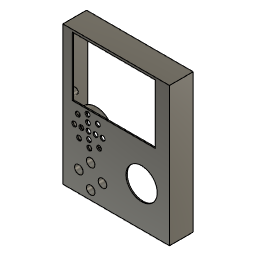
front2 (Autodesk Fusion 360 design; units mm, degrees)
Autodesk Fusion 360 part; units mm, degrees
sketch "Sketch1" plane through (0, 0, 0) normal (0, 1, 0) x (1, 0, 0)
  line L0 (-88, -115.2) -> (-2, -115.2)
  line L1 (-2, -115.2) -> (-2, -65.2)
  line L2 (-2, -65.2) -> (-88, -65.2)
  line L3 (-88, -65.2) -> (-88, -115.2)
  line L4 (-12, -115.2) -> (-82, -115.2)
  line L5 (-82, -115.2) -> (-82, -65.2)
  line L6 (-82, -65.2) -> (-12, -65.2)
  line L7 (-12, -65.2) -> (-12, -115.2)
  circle A0 centre (-85, -112.2) radius 1.5
  circle A1 centre (-85, -68.2) radius 1.5
  circle A2 centre (-8.8, -112.2) radius 1.5
  circle A3 centre (-8.8, -68.2) radius 1.5
  line L8 (-72, -33) -> (-61, -33)
  line L9 (-61, -33) -> (-61, -22)
  line L10 (-61, -22) -> (-72, -22)
  line L11 (-72, -22) -> (-72, -33)
  line L12 (-62, -23) -> (-51, -23)
  line L13 (-51, -23) -> (-51, -12)
  line L14 (-51, -12) -> (-62, -12)
  line L15 (-62, -12) -> (-62, -23)
  line L16 (-61, -13) -> (-72, -13)
  line L17 (-72, -13) -> (-72, -2)
  line L18 (-72, -2) -> (-61, -2)
  line L19 (-61, -2) -> (-61, -13)
  line L20 (-71, -23) -> (-82, -23)
  line L21 (-82, -23) -> (-82, -12)
  line L22 (-82, -12) -> (-71, -12)
  line L23 (-71, -12) -> (-71, -23)
  line L24 (-61, -22) -> (-52, -22)
  line L25 (-52, -22) -> (-52, -13)
  line L26 (-52, -13) -> (-61, -13)
  line L27 (-61, -13) -> (-61, -22)
  line L28 (-71, -23) -> (-62, -23)
  line L29 (-62, -23) -> (-62, -32)
  line L30 (-62, -32) -> (-71, -32)
  line L31 (-71, -32) -> (-71, -23)
  line L32 (-72, -22) -> (-81, -22)
  line L33 (-81, -22) -> (-81, -13)
  line L34 (-81, -13) -> (-72, -13)
  line L35 (-72, -13) -> (-72, -22)
  line L36 (-71, -12) -> (-62, -12)
  line L37 (-62, -12) -> (-62, -3)
  line L38 (-62, -3) -> (-71, -3)
  line L39 (-71, -3) -> (-71, -12)
  circle A4 centre (-66.5, -7.5) radius 3.6
  circle A5 centre (-76.5, -17.5) radius 3.6
  circle A6 centre (-56.5, -17.5) radius 3.6
  circle A7 centre (-66.5, -27.5) radius 3.6
  circle A8 centre (-73.5, -10.5) radius 1.5
  circle A9 centre (-59.5, -24.5) radius 1.5
  circle A10 centre (-59.5, -24.5) radius 2.5
  circle A11 centre (-73.5, -10.5) radius 2.5
  line L40 (-73.5048, -8) -> (-72, -8)
  line L41 (-72, -8) -> (-72, -8.5)
  line L42 (-72, -8.5) -> (-73.5048, -8.5)
  line L43 (-73.5048, -8.5) -> (-73.5048, -8)
  line L44 (-76, -10.5053) -> (-75.5, -10.5053)
  line L45 (-75.5, -10.5053) -> (-75.5, -12)
  line L46 (-75.5, -12) -> (-76, -12)
  line L47 (-76, -12) -> (-76, -10.5053)
  line L48 (-57, -24.4959) -> (-57.5, -24.4959)
  line L49 (-57.5, -24.4959) -> (-57.5, -23)
  line L50 (-57.5, -23) -> (-57, -23)
  line L51 (-57, -23) -> (-57, -24.4959)
  line L52 (-59.4955, -27) -> (-61, -27)
  line L53 (-61, -27) -> (-61, -26.5)
  line L54 (-61, -26.5) -> (-59.4955, -26.5)
  line L55 (-59.4955, -26.5) -> (-59.4955, -27)
  circle A12 centre (-23.5, -33.6) radius 13.2
  circle A13 centre (-68.4, -49.6) radius 14.1
  circle A14 centre (-68.4, -49.6) radius 14.6
  circle A15 centre (-68.4, -49.6) radius 2
  circle A16 centre (-69.1779, -61.5748) radius 2
  circle A17 centre (-68.8197, -55.5853) radius 2
  circle A18 centre (-60.4826, -58.6175) radius 2
  circle A19 centre (-56.4253, -50.3779) radius 2
  circle A20 centre (-59.3825, -41.6826) radius 2
  circle A21 centre (-67.6221, -37.6252) radius 2
  circle A22 centre (-76.3174, -40.5825) radius 2
  circle A23 centre (-80.3748, -48.8221) radius 2
  circle A24 centre (-77.4175, -57.5174) radius 2
  circle A25 centre (-62.4147, -50.0197) radius 2
  circle A26 centre (-67.9803, -43.6147) radius 2
  circle A27 centre (-74.3853, -49.1803) radius 2
  circle A28 centre (-51.3037, -49.9525) radius 2.5
  circle A29 centre (-51.3037, -49.9525) radius 1.5
  circle A30 centre (-85.5, -49.572) radius 2.5
  circle A31 centre (-85.5, -49.572) radius 1.5
  line L56 (-85.6266, -52.0687) -> (-83, -52.0687)
  line L57 (-83, -52.0687) -> (-83, -49.5761)
  line L58 (-83, -49.5761) -> (-85.6266, -49.5761)
  line L59 (-85.6266, -49.5761) -> (-85.6266, -52.0687)
  line L60 (-82.7898, -52.0687) -> (-83, -52.0687)
  line L61 (-83, -52.0687) -> (-83, -49.5761)
  line L62 (-83, -49.5761) -> (-82.7898, -49.5761)
  line L63 (-82.7898, -49.5761) -> (-82.7898, -52.0687)
  line L64 (-85.3581, -47.076) -> (-82.7898, -47.076)
  line L65 (-82.7898, -47.076) -> (-82.7898, -49.5761)
  line L66 (-82.7898, -49.5761) -> (-85.3581, -49.5761)
  line L67 (-85.3581, -49.5761) -> (-85.3581, -47.076)
  line L68 (-51.4135, -52.4501) -> (-53.8031, -52.4501)
  line L69 (-53.8031, -52.4501) -> (-53.8031, -49.901)
  line L70 (-53.8031, -49.901) -> (-51.4135, -49.901)
  line L71 (-51.4135, -49.901) -> (-51.4135, -52.4501)
  line L72 (-53.8031, -49.901) -> (-51.1807, -49.901)
  line L73 (-51.1807, -49.901) -> (-51.1807, -47.4555)
  line L74 (-51.1807, -47.4555) -> (-53.8031, -47.4555)
  line L75 (-53.8031, -47.4555) -> (-53.8031, -49.901)
  line L76 (-53.9584, -47.4555) -> (-53.8031, -47.4555)
  line L77 (-53.8031, -47.4555) -> (-53.8031, -49.901)
  line L78 (-53.8031, -49.901) -> (-53.9584, -49.901)
  line L79 (-53.9584, -49.901) -> (-53.9584, -47.4555)
  line L80 (-54.0809, -52.4501) -> (-53.8031, -52.4501)
  line L81 (-53.8031, -52.4501) -> (-53.8031, -49.901)
  line L82 (-53.8031, -49.901) -> (-54.0809, -49.901)
  line L83 (-54.0809, -49.901) -> (-54.0809, -52.4501)
  line L84 (-90, -117.2) -> (0, -117.2)
  line L85 (0, -117.2) -> (0, 0)
  line L86 (0, 0) -> (-90, 0)
  line L87 (-90, 0) -> (-90, -117.2)
  line L88 (-89, -116.2) -> (-1, -116.2)
  line L89 (-1, -116.2) -> (-1, -1)
  line L90 (-1, -1) -> (-89, -1)
  line L91 (-89, -1) -> (-89, -116.2)
  circle A32 centre (-85, -112.2) radius 2.5
  circle A33 centre (-85, -68.2) radius 2.5
  circle A34 centre (-8.8, -68.2) radius 2.5
  circle A35 centre (-8.8, -112.2) radius 2.5
  dimension "d1" = 86
  dimension "d2" = 50
  dimension "d3" = 70
  dimension "d4" = 50
  dimension "d5" = 10
  dimension "d6" = 3
  dimension "d7" = 3
  dimension "d8" = 3
  dimension "d9" = 3
  dimension "d10" = 3
  dimension "d11" = 3
  dimension "d12" = 3
  dimension "d13" = 3
  dimension "d14" = 6.8
  dimension "d15" = 3
  dimension "d16" = 6.8
  dimension "d17" = 3
  dimension "d18" = 11
  dimension "d19" = 11
  dimension "d20" = 11
  dimension "d21" = 11
  dimension "d22" = 11
  dimension "d23" = 11
  dimension "d24" = 11
  dimension "d25" = 11
  dimension "d26" = 1
  dimension "d27" = 1
  dimension "d28" = 1
  dimension "d29" = 1
  dimension "d30" = 1
  dimension "d31" = 1
  dimension "d32" = 9
  dimension "d33" = 9
  dimension "d34" = 9
  dimension "d35" = 9
  dimension "d36" = 9
  dimension "d37" = 9
  dimension "d38" = 9
  dimension "d39" = 9
  dimension "d40" = 7.2
  dimension "d41" = 7.2
  dimension "d42" = 7.2
  dimension "d43" = 7.2
  dimension "d44" = 4.5
  dimension "d45" = 4.5
  dimension "d46" = 4.5
  dimension "d47" = 4.5
  dimension "d48" = 4.5
  dimension "d49" = 4.5
  dimension "d50" = 4.5
  dimension "d51" = 4.5
  dimension "d52" = 3
  dimension "d53" = 3
  dimension "d54" = 1.5
  dimension "d55" = 1.5
  dimension "d56" = 1.5
  dimension "d57" = 1.5
  dimension "d58" = 5
  dimension "d59" = 5
  dimension "d60" = 26.4
  dimension "d61" = 28.2
  dimension "d62" = 29.2
  dimension "d63" = 4
  dimension "d64" = 4
  dimension "d65" = 12
  dimension "d66" = 4
  dimension "d67" = 6
  dimension "d69" = 360
  dimension "d71" = 360
  dimension "d72" = 5
  dimension "d73" = 3
  dimension "d74" = 5
  dimension "d75" = 3
  dimension "d76" = 17.1
  dimension "d77" = 17.0964
  dimension "d78" = 15.6
  dimension "d79" = 2.5
  dimension "d80" = 16.6
  dimension "d81" = 7.4
  dimension "d83" = 27.5
  dimension "d85" = 31.6
  dimension "d86" = 2
  dimension "d87" = 2
  dimension "d88" = 2
  dimension "d89" = 2
  dimension "d90" = 1
  dimension "d91" = 1
  dimension "d92" = 1
  dimension "d93" = 1
  dimension "d98" = 5
  dimension "d99" = 5
  dimension "d100" = 5
  dimension "d101" = 5
  constraint horizontal L0
  constraint vertical L1
  constraint horizontal L2
  constraint vertical L3
  constraint horizontal L4
  constraint vertical L5
  constraint horizontal L6
  constraint vertical L7
  constraint coincident L0 L4.start
  constraint horizontal L8
  constraint vertical L9
  constraint horizontal L10
  constraint vertical L11
  constraint horizontal L12
  constraint vertical L13
  constraint horizontal L14
  constraint vertical L15
  constraint horizontal L16
  constraint vertical L17
  constraint horizontal L18
  constraint vertical L19
  constraint horizontal L20
  constraint vertical L21
  constraint horizontal L22
  constraint vertical L23
  constraint horizontal L24
  constraint vertical L25
  constraint horizontal L26
  constraint vertical L27
  constraint horizontal L28
  constraint vertical L29
  constraint horizontal L30
  constraint vertical L31
  constraint horizontal L32
  constraint vertical L33
  constraint horizontal L34
  constraint vertical L35
  constraint horizontal L36
  constraint vertical L37
  constraint horizontal L38
  constraint vertical L39
  constraint concentric A9 A10
  constraint concentric A8 A11
  constraint horizontal L40
  constraint vertical L41
  constraint horizontal L42
  constraint vertical L43
  constraint coincident A11 L41.end
  constraint coincident L17 L41.end
  constraint coincident A11 L40.start
  constraint horizontal L44
  constraint vertical L45
  constraint horizontal L46
  constraint vertical L47
  constraint coincident A11 L45.end
  constraint coincident L22 L45.end
  constraint coincident A11 L44.start
  constraint horizontal L48
  constraint vertical L49
  constraint horizontal L50
  constraint vertical L51
  constraint coincident L12 L49.end
  constraint coincident A10 L49.end
  constraint coincident A10 L48.start
  constraint horizontal L52
  constraint vertical L53
  constraint horizontal L54
  constraint vertical L55
  constraint coincident A10 L53.end
  constraint coincident L9 L53.end
  constraint coincident A10 L52.start
  constraint concentric A13 A14
  constraint concentric A13 A15
  constraint concentric A28 A29
  constraint tangent A14 A28
  constraint concentric A30 A31
  constraint tangent A14 A30
  constraint horizontal L56
  constraint vertical L57
  constraint horizontal L58
  constraint vertical L59
  constraint coincident A30 L57.end
  constraint coincident A14 L57.end
  constraint coincident A30 L56.start
  constraint horizontal L60
  constraint vertical L61
  constraint horizontal L62
  constraint vertical L63
  constraint coincident A14 L60.start
  constraint horizontal L64
  constraint vertical L65
  constraint horizontal L66
  constraint vertical L67
  constraint coincident A30 L64.start
  constraint horizontal L68
  constraint vertical L69
  constraint horizontal L70
  constraint vertical L71
  constraint coincident A28 L69.end
  constraint coincident A14 L69.end
  constraint coincident A28 L68.start
  constraint horizontal L72
  constraint vertical L73
  constraint horizontal L74
  constraint vertical L75
  constraint coincident A28 L73.end
  constraint horizontal L76
  constraint vertical L77
  constraint horizontal L78
  constraint vertical L79
  constraint coincident A14 L76.start
  constraint horizontal L80
  constraint vertical L81
  constraint horizontal L82
  constraint vertical L83
  constraint coincident A14 L80.start
  constraint coincident L68.end L80
  constraint coincident L74.end L76
  constraint coincident L56.end L60
  constraint horizontal L84
  constraint vertical L85
  constraint horizontal L86
  constraint vertical L87
  constraint horizontal L88
  constraint vertical L89
  constraint horizontal L90
  constraint vertical L91
  constraint concentric A0 A32
  constraint concentric A1 A33
  constraint concentric A3 A34
  constraint concentric A2 A35
  constraint coincident L85.end L86.start
  measures "d1" distance of L0.start L0.end
  measures "d2" distance of L0.start L2.end
  measures "d3" distance of L4.start L4.end
  measures "d4" distance of L4.start L6.end
  measures "d5" distance of L1 L7
  measures "d6" diameter of A0
  measures "d7" diameter of A1
  measures "d8" diameter of A2
  measures "d9" diameter of A3
  measures "d10" distance of L3 A1.centre
  measures "d11" distance of L2 A1.centre
  measures "d12" distance of L3 A0.centre
  measures "d13" distance of L0 A0.centre
  measures "d14" distance of L1 A2.centre
  measures "d15" distance of L0 A2.centre
  measures "d16" distance of L1 A3.centre
  measures "d17" distance of L2 A3.centre
  measures "d18" distance of L8.start L8.end
  measures "d19" distance of L8.start L10.end
  measures "d20" distance of L12.start L12.end
  measures "d21" distance of L12.start L14.end
  measures "d22" distance of L16.start L16.end
  measures "d23" distance of L16.start L18.end
  measures "d24" distance of L20.start L20.end
  measures "d25" distance of L20.start L22.end
  measures "d26" distance of L16 L22
  measures "d27" distance of L17 L23
  measures "d28" distance of L15 L19
  measures "d29" distance of L14 L16
  measures "d30" distance of L10 L12
  measures "d31" distance of L9 L15
  measures "d32" distance of L9.end L24.end
  measures "d33" distance of L9.end L16.start
  measures "d34" distance of L20.start L12.start
  measures "d35" distance of L20.start L30.end
  measures "d36" distance of L10.end L32.end
  measures "d37" distance of L10.end L16.end
  measures "d38" distance of L22.end L14.end
  measures "d39" distance of L22.end L38.end
  measures "d40" diameter of A4
  measures "d41" diameter of A5
  measures "d42" diameter of A6
  measures "d43" diameter of A7
  measures "d44" distance of L39 A4.centre
  measures "d45" distance of L38 A4.centre
  measures "d46" distance of L26 A6.centre
  measures "d47" distance of L25 A6.centre
  measures "d48" distance of L34 A5.centre
  measures "d49" distance of L35 A5.centre
  measures "d50" distance of L29 A7.centre
  measures "d51" distance of L28 A7.centre
  measures "d52" diameter of A8
  measures "d53" diameter of A9
  measures "d54" distance of L22 A8.centre
  measures "d55" distance of L17 A8.centre
  measures "d56" distance of L12 A9.centre
  measures "d57" distance of L9 A9.centre
  measures "d58" diameter of A10
  measures "d59" diameter of A11
  measures "d60" diameter of A12
  measures "d61" diameter of A13
  measures "d62" diameter of A14
  measures "d63" diameter of A15
  measures "d64" diameter of A16
  measures "d65" distance of A13.centre A16.centre
  measures "d66" diameter of A17
  measures "d67" distance of A13.centre A17.centre
  measures "d72" diameter of A28
  measures "d73" diameter of A29
  measures "d74" diameter of A30
  measures "d75" diameter of A31
  measures "d76" horizontal distance of A13.centre A30.centre
  measures "d77" horizontal distance of A13.centre A28.centre
  measures "d78" distance of L2 A13.centre
  measures "d79" distance of L3 A30.centre
  measures "d80" distance of L8 A13.centre
  measures "d81" distance of L9 A13.centre
  measures "d83" distance of L13 A12.centre
  measures "d85" distance of L2 A12.centre
  measures "d86" distance of L18 L86
  measures "d87" distance of L3 L87
  measures "d88" distance of L4 L84
  measures "d89" distance of L1 L85
  measures "d90" distance of L85 L89
  measures "d91" distance of L84 L88
  measures "d92" distance of L87 L91
  measures "d93" distance of L86 L90
  measures "d98" diameter of A32
  measures "d99" diameter of A33
  measures "d100" diameter of A34
  measures "d101" diameter of A35
extrude "Extrude1" add sketch "Sketch1" against normal blind 1 contours L0 L2 L3 L5 | L0 L1 L2 L7 | A0 | A1 | A2 | A3 | L8 L9 L11 L20 L29 L30 L31 A10 L53 | L17 A11 L40 L41 | L9 A10 L52 L53 | L11 L20 L21 L22 L32 L33 L34 A11 L46 | L10 L11 L20 L23 | L10 L16 L23 L35 | L32 L33 L34 L35 | L10 L15 L23 L28 | L28 L29 L30 L31 | L9 L12 A10 | A10 L54 L55 | L9 L12 A9 A10 L48 L49 L54 L55 | L10 L15 L16 L23 | L16 L17 L22 L23 A11 | L17 L34 A11 | L9 L10 L12 L15 A10 | L12 L29 A10 | L9 L12 A9 | A9 | L10 L15 L16 L27 | L15 L16 L23 L36 | L17 L22 A11 | L17 L22 A11 | L9 L12 A10 | L22 A11 L46 L47 | L9 L12 A10 | A10 L48 L49 | L12 A10 L50 L51 | L9 L24 A10 | L24 L25 L26 L27 | L14 L15 L16 L19 | L36 L37 L38 L39 | L22 L39 A11 | L17 L22 A8 | L17 L22 A11 | L17 L22 A8 A11 L42 L43 L44 L45 | A11 L44 L45 | L12 L13 L14 L19 L24 L25 L26 A10 L50 | L14 L17 L18 L19 L37 L38 L39 A11 L41 | A8 | A11 L42 L43 | A13 | A14 A30 L62 L65 L66 | A14 A30 L64 L65 | A14 A30 A31 L58 L66 L67 | A14 L62 L63 L66 | A28 A29 L70 L72 L73 | A30 A31 L59 L67 | A30 L56 L57 L61 | A14 L57 L60 L61 | A30 A31 L58 L59 L66 | A14 L63 L65 L79 L82 L83 | A31 L58 L66 L67 | A31 L58 L59 L66 | A14 L75 L76 L77 | A14 L75 L77 L78 L79 L82 | A31 L58 L59 L67 | A14 L78 L82 L83 | A28 A29 L70 L71 L72 | A14 L69 L80 L81 | A28 A29 L71 L73 | A14 A28 L74 L75 L77 | A14 L75 L77 | A28 L68 L69 L81 | A29 L70 L71 L72 | A29 L70 L72 L73 | A29 L71 L72 L73 | L84 L85 L86 L87 | L88 L89 L90 L91 | A32 | A33 | A34 | A35
extrude "Extrude2" add sketch "Sketch1" along normal blind 5.5 contours A14 A30 L62 L65 L66 | A14 A30 L64 L65 | A14 A30 A31 L58 L66 L67 | A14 L62 L63 L66 | A28 A29 L70 L72 L73 | A30 A31 L59 L67 | A30 L56 L57 L61 | A14 L57 L60 L61 | A30 A31 L58 L59 L66 | A14 L63 L65 L79 L82 L83 | A14 L75 L76 L77 | A14 L75 L77 L78 L79 L82 | A14 L78 L82 L83 | A28 A29 L70 L71 L72 | A14 L69 L80 L81 | A28 A29 L71 L73 | A14 A28 L74 L75 L77 | A14 L75 L77 | A28 L68 L69 L81
extrude "Extrude3" add sketch "Sketch1" along normal blind 4.5 contours A32 | A33 | A34 | A35
extrude "Extrude4" add sketch "Sketch1" along normal blind 6.5 contours L32 L33 L34 L35 | L28 L29 L30 L31 | L24 L25 L26 L27 | L36 L37 L38 L39
extrude "Extrude5" add sketch "Sketch1" along normal blind 14.5 contours L8 L9 L11 L20 L29 L30 L31 A10 L53 | L17 A11 L40 L41 | L9 A10 L52 L53 | L11 L20 L21 L22 L32 L33 L34 A11 L46 | L10 L11 L20 L23 | L10 L16 L23 L35 | L10 L15 L23 L28 | L9 L12 A10 | A10 L54 L55 | L9 L12 A9 A10 L48 L49 L54 L55 | L16 L17 L22 L23 A11 | L17 L34 A11 | L9 L10 L12 L15 A10 | L12 L29 A10 | L9 L12 A9 | L10 L15 L16 L27 | L15 L16 L23 L36 | L17 L22 A11 | L17 L22 A11 | L9 L12 A10 | L22 A11 L46 L47 | L9 L12 A10 | A10 L48 L49 | L12 A10 L50 L51 | L9 L24 A10 | L14 L15 L16 L19 | L22 L39 A11 | L17 L22 A8 | L17 L22 A11 | L17 L22 A8 A11 L42 L43 L44 L45 | A11 L44 L45 | L12 L13 L14 L19 L24 L25 L26 A10 L50 | L14 L17 L18 L19 L37 L38 L39 A11 L41 | A11 L42 L43
extrude "Extrude6" cut 4 faces at (-56.5897, 6.5, 21.6966) (-66.4103, 6.5, 31.6966) (-76.5897, 6.5, 21.6966) (-66.5897, 6.5, 3.3034) along direction (0, -1, 0) blind 1
extrude "Extrude7" add sketch "Sketch1" along normal blind 19 contours L84 L85 L86 L87
equation "d81 = 11 mm - 3.6 mm"
equation "d83 = 6 mm + 8.3 mm + 13.2 mm"
equation "d106 = 5.50 mm + 9 mm"
